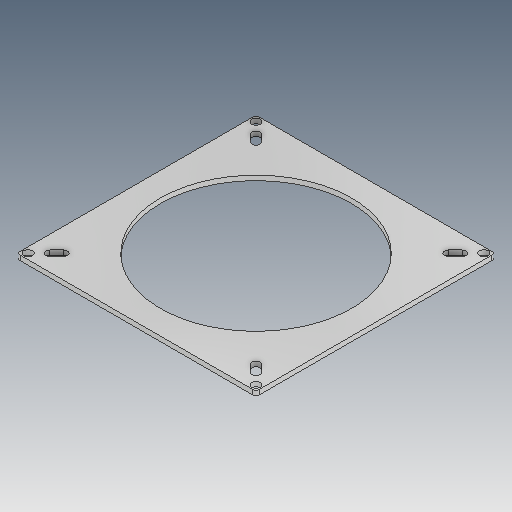
# Autodesk Inventor part: 150mm_Bearing_Plate
Saved by Autodesk Inventor 2020.3 (Build 243373000, 373)
## iProperties
Created: 2021-09-01
Part Number: 150mm_Bearing_Plate
Material: Aluminum 6061
Document SubType Name: Modeling
Designer: justi
Density: 2.7 g/cm^3
Appearance: Aluminum - Dark
Mass: 88.2354 g
Surface Area: 252.47 cm^2
Volume: 32.6798 cm^3
Author: justi
Autodesk Inventor part; units mm, degrees
ref_plane "YZ Plane" through (0, 0, 0) normal (1, 0, 0) x (0, 1, 0)
ref_plane "XZ Plane" through (0, 0, 0) normal (0, 1, 0) x (-1, 0, 0)
ref_plane "XY Plane" through (0, 0, 0) normal (0, 0, 1) x (1, 0, 0)
sketch "Sketch1" plane through (0, 0, 0) normal (0, 1, 0) x (-1, 0, 0)
  line L0 (-75, 75) -> (75, 75)
  line L1 (75, 75) -> (75, -75)
  line L2 (75, -75) -> (-75, -75)
  line L3 (-75, -75) -> (-75, 75)
  line L4 (-75, 75) -> (75, -75) construction
  line L5 (75, 75) -> (-75, -75) construction
  circle A0 centre (0, 0) radius 60
  line L6 (-62.5, 62.5) -> (62.5, 62.5) construction
  line L7 (62.5, 62.5) -> (62.5, -62.5) construction
  line L8 (62.5, -62.5) -> (-62.5, -62.5) construction
  line L9 (-62.5, -62.5) -> (-62.5, 62.5) construction
  line L10 (-62.5, 62.5) -> (62.5, -62.5) construction
  line L11 (62.5, 62.5) -> (-62.5, -62.5) construction
  circle A1 centre (62.5, 62.5) radius 2.5
  circle A2 centre (62.5, -62.5) radius 2.5
  circle A3 centre (-62.5, 62.5) radius 2.5
  circle A4 centre (-62.5, -62.5) radius 2.5
  line L12 (64.6213, -64.6213) -> (60.3787, -60.3787) construction
  line L13 (62.8536, -66.3891) -> (58.6109, -62.1464)
  line L14 (62.1464, -58.6109) -> (66.3891, -62.8536)
  arc A5 (62.8536, -66.3891) -> (66.3891, -62.8536) centre (64.6213, -64.6213) ccw
  arc A6 (62.1464, -58.6109) -> (58.6109, -62.1464) centre (60.3787, -60.3787) ccw
  line L15 (-64.6213, -64.6213) -> (-60.3787, -60.3787) construction
  line L16 (-62.8536, -66.3891) -> (-58.6109, -62.1464)
  line L17 (-62.1464, -58.6109) -> (-66.3891, -62.8536)
  arc A7 (-66.3891, -62.8536) -> (-62.8536, -66.3891) centre (-64.6213, -64.6213) ccw
  arc A8 (-58.6109, -62.1464) -> (-62.1464, -58.6109) centre (-60.3787, -60.3787) ccw
  line L18 (-64.6213, 64.6213) -> (-60.3787, 60.3787) construction
  line L19 (-62.8536, 66.3891) -> (-58.6109, 62.1464)
  line L20 (-62.1464, 58.6109) -> (-66.3891, 62.8536)
  arc A9 (-62.8536, 66.3891) -> (-66.3891, 62.8536) centre (-64.6213, 64.6213) ccw
  arc A10 (-62.1464, 58.6109) -> (-58.6109, 62.1464) centre (-60.3787, 60.3787) ccw
  line L21 (64.6213, 64.6213) -> (60.3787, 60.3787) construction
  line L22 (62.8536, 66.3891) -> (58.6109, 62.1464)
  line L23 (62.1464, 58.6109) -> (66.3891, 62.8536)
  arc A11 (66.3891, 62.8536) -> (62.8536, 66.3891) centre (64.6213, 64.6213) ccw
  arc A12 (58.6109, 62.1464) -> (62.1464, 58.6109) centre (60.3787, 60.3787) ccw
  dimension "d0" = 150
  dimension "d1" = 150
  dimension "d2" = 120
  dimension "d3" = 125
  dimension "d4" = 5
  dimension "d5" = 5
  dimension "d6" = 5
  dimension "d7" = 5
  dimension "d21" = 3
  dimension "d22" = 3
  dimension "d23" = 3
  dimension "d24" = 3
  constraints: 56 end point, 16 point on circle, 16 tangent, 13 centre point, 8 midpoint, 8 parallel, 5 coincident, 5 point on line, 2 horizontal, 2 perpendicular
  measures "d0" distance of L1.end L2.end
  measures "d1" distance of L0.end L1.end
  measures "d2" diameter of A0
  measures "d3" distance of L7.end L8.end
  measures "d4" diameter of A1
  measures "d5" diameter of A2
  measures "d6" diameter of A3
  measures "d7" diameter of A4
  measures "d21" distance of A2.centre L12.end
  measures "d22" distance of A4.centre L15.end
  measures "d23" distance of A3.centre L18.end
  measures "d24" distance of A1.centre L21.end
extrude "Extrusion1" add sketch "Sketch1" along normal blind 3
sketch "Sketch2" plane through (0, 0, 0) normal (0, -1, 0) x (1, 0, 0)
  line L0 (-71.5, -71.5) -> (71.5, -71.5)
  line L1 (71.5, -71.5) -> (71.5, 71.5)
  line L2 (71.5, 71.5) -> (-71.5, 71.5)
  line L3 (-71.5, 71.5) -> (-71.5, -71.5)
  line L4 (-71.5, -71.5) -> (71.5, 71.5) construction
  line L5 (71.5, -71.5) -> (-71.5, 71.5) construction
  point P0 (0, 0)
  dimension "d11" = 143
  dimension "d19" = 143
  constraints: 12 end point, 2 midpoint, 2 parallel, 1 horizontal, 1 perpendicular
  measures "d11" distance of L2.end L1.end
  measures "d19" distance of L2.end L0.start
hole "Hole1" at (-71.5, 0, 71.5) at (71.5, 0, 71.5) at (71.5, 0, -71.5) at (-71.5, 0, -71.5) direction (0, 1, 0) diameter 5.5 depth 6 tip angle 118
fillet "Fillet2" radius 2 4 edges at (-75, 1.5, 75) (75, 1.5, 75) (-75, 1.5, -75) (75, 1.5, -75)
equation "\"d8\" = d24"
body "Solid1"
